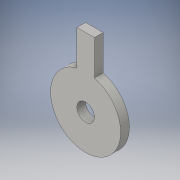
# Autodesk Inventor part: spinnything
Saved by Autodesk Inventor 2016 (Build 200138000, 138)
## iProperties
Created: 2015-12-12
Part Number: spinnything
Material: Generic
Document SubType Name: Modeling
Designer: Louis
Density: 1 g/cm^3
Appearance: Default
Author: Louis
Autodesk Inventor part; units mm, degrees
ref_plane "YZ Plane" through (0, 0, 0) normal (1, 0, 0) x (0, 1, 0)
ref_plane "XZ Plane" through (0, 0, 0) normal (0, 1, 0) x (-1, 0, 0)
ref_plane "XY Plane" through (0, 0, 0) normal (0, 0, 1) x (1, 0, 0)
sketch "Sketch1" plane through (0, 0, 0) normal (0, 0, 1) x (1, 0, 0)
  circle A0 centre (0, 0) radius 3.175
  circle A1 centre (0, 0) radius 12.7
  line L0 (-3.175, 12.2967) -> (3.175, 12.2967)
  line L1 (-3.175, 12.2967) -> (3.175, 12.2967)
  line L2 (3.175, 12.2967) -> (3.175, 24.9967)
  line L3 (3.175, 24.9967) -> (-3.175, 24.9967)
  line L4 (-3.175, 24.9967) -> (-3.175, 12.2967)
  dimension "d0" = 6.35
  dimension "d1" = 25.4
  dimension "d2" = 6.35
  dimension "d3" = 12.7
  dimension "d4" = 6.35
  constraints: 10 end point, 2 centre point, 2 coincident, 2 horizontal, 2 parallel, 2 point on circle, 1 perpendicular
  measures "d0" diameter of A0
  measures "d1" diameter of A1
  measures "d2" distance of L0.start L0.end
  measures "d3" distance of L2.end L1.end
  measures "d4" distance of L2.end L3.end
extrude "Extrusion1" add sketch "Sketch1" along normal blind 3.175
body "Solid1"
